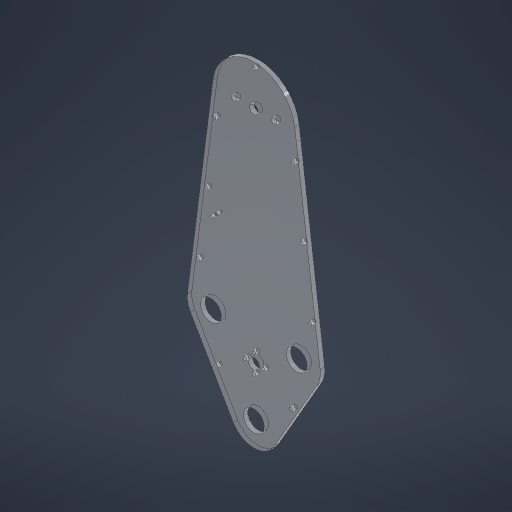
# Autodesk Inventor part: 2ELO
Saved by Autodesk Inventor 2025.2 (Build 292293000, 293)
## iProperties
Created: 2025-05-02
Part Number: 2ELO
Material: Generic
Document SubType Name: Modeling
Designer: Nelson
Density: 1 g/cm^3
Appearance: Polycarbonate - Clear
Author: Nelson
Autodesk Inventor part; units mm, degrees
ref_plane "YZ Plane" through (0, 0, 0) normal (1, 0, 0) x (0, 1, 0)
ref_plane "XZ Plane" through (0, 0, 0) normal (0, 1, 0) x (-1, 0, 0)
ref_plane "XY Plane" through (0, 0, 0) normal (0, 0, 1) x (1, 0, 0)
sketch "Sketch1" plane through (0, 0, 0) normal (0, 0, 1) x (1, 0, 0)
  line L0 (0, 0) -> (0, 200) construction
  arc A0 (37.1934, 204.7857) -> (-37.1934, 204.7857) centre (0, 200) ccw
  line L1 (0, 200) -> (-18.25, 200) construction
  circle A1 centre (-18.25, 200) radius 2.5
  line L2 (0, 200) -> (18.25, 200) construction
  circle A2 centre (18.25, 200) radius 2.5
  circle A3 centre (0, 0) radius 15 construction
  line L3 (37.1934, 204.7857) -> (59.7122, 29.7756)
  line L4 (-37.1934, 204.7857) -> (-59.9286, 28.0941)
  line L5 (48.4528, 117.2807) -> (43.4937, 116.6426) construction
  line L6 (51.1509, 57.1332) -> (35.8365, 176.152) construction
  circle A4 centre (35.8365, 176.152) radius 1.5
  circle A5 centre (51.1509, 57.1332) radius 1.5
  circle A6 centre (43.4937, 116.6426) radius 1.5
  line L7 (0, 237.5) -> (0, 232.5) construction
  circle A7 centre (0, 232.5) radius 1.5
  circle A8 centre (-35.8365, 176.152) radius 1.5
  circle A9 centre (-43.4937, 116.6426) radius 1.5
  circle A10 centre (-51.1509, 57.1332) radius 1.5
  circle A11 centre (0, 200) radius 4
  circle A12 centre (0, 0) radius 45 construction
  circle A13 centre (0, -45) radius 9.5
  circle A14 centre (0, -45) radius 14.5 construction
  circle A15 centre (0, -59.5) radius 2.25 construction
  circle A16 centre (14.5, -45) radius 2.25 construction
  circle A17 centre (0, -30.5) radius 2.25 construction
  circle A18 centre (-14.5, -45) radius 2.25 construction
  circle A19 centre (0, -45) radius 21.5 construction
  circle A20 centre (38.9711, 22.5) radius 21.5 construction
  circle A21 centre (51.5285, 29.75) radius 2.25 construction
  circle A22 centre (46.2211, 9.9426) radius 2.25 construction
  circle A23 centre (31.7211, 35.0574) radius 2.25 construction
  circle A24 centre (26.4138, 15.25) radius 2.25 construction
  circle A25 centre (38.9711, 22.5) radius 9.5
  circle A26 centre (-38.9711, 22.5) radius 21.5 construction
  circle A27 centre (-51.5285, 29.75) radius 2.25 construction
  circle A28 centre (-31.7211, 35.0574) radius 2.25 construction
  circle A29 centre (-46.2211, 9.9426) radius 2.25 construction
  circle A30 centre (-26.4138, 15.25) radius 2.25 construction
  circle A31 centre (-38.9711, 22.5) radius 9.5
  line L8 (-18.6195, -55.75) -> (-57.5907, 11.75)
  line L9 (18.6195, -55.75) -> (57.5907, 11.75)
  line L10 (48.4528, 117.2807) -> (48.4528, 23.0901) construction
  line L11 (59.7122, 29.7756) -> (60.2953, 25.2438)
  line L12 (48.4528, 23.0901) -> (48.4528, -26.9099) construction
  line L13 (48.4528, -26.9099) -> (38.566, -21.2018) construction
  line L14 (38.566, -21.2018) -> (34.2359, -18.7018) construction
  circle A32 centre (34.2359, -18.7018) radius 1.5
  circle A33 centre (-34.2359, -18.7018) radius 1.5
  arc A34 (57.5907, 11.75) -> (60.2953, 25.2438) centre (38.9711, 22.5) ccw
  arc A35 (-60.2953, 25.2438) -> (-57.5907, 11.75) centre (-38.9711, 22.5) ccw
  arc A36 (-18.6195, -55.75) -> (18.6195, -55.75) centre (0, -45) ccw
  line L15 (38.9711, 22.5) -> (53.4711, 22.5) construction
  line L16 (-59.9286, 28.0941) -> (-60.2953, 25.2438)
  circle A37 centre (0, 0) radius 5.1
  line L17 (0, 0) -> (0, -8) construction
  circle A38 centre (0, -8) radius 1.75
  circle A39 centre (8, 0) radius 1.75
  circle A40 centre (0, 8) radius 1.75
  circle A41 centre (-8, 0) radius 1.75
  line L18 (0, 200) -> (0, 135) construction
  line L19 (0, 135) -> (-52.9913, 82.0087) construction
  line L20 (-52.9913, 82.0087) -> (-38.8492, 96.1508) construction
  circle A42 centre (-38.8492, 96.1508) radius 1.1
  line L21 (-38.8492, 96.1508) -> (-33.8994, 101.1006) construction
  circle A43 centre (-33.8994, 101.1006) radius 1.1
  dimension "d84" = 90
  dimension "d86" = 29
  dimension "d58" = 200
  dimension "d59" = 75
  dimension "d60" = 18.25
  dimension "d61" = 5
  dimension "d62" = 30
  dimension "d63" = 5
  dimension "d64" = 120
  dimension "d65" = 3
  dimension "d66" = 3
  dimension "d67" = 3
  dimension "d68" = 5
  dimension "d69" = 3
  dimension "d70" = 8
  dimension "d85" = 19
  dimension "d87" = 4.5
  dimension "d88" = 45
  dimension "d89" = 14.5
  dimension "d90" = 14.5
  dimension "d91" = 360
  dimension "d92" = 43
  dimension "d93" = 360
  dimension "d94" = 94.1906
  dimension "d95" = 50
  dimension "d96" = 5
  dimension "d97" = 3
  dimension "d103" = 10.2
  dimension "d104" = 8
  dimension "d105" = 3.5
  dimension "d108" = 360
  dimension "d110" = 65
  dimension "d111" = 45
  dimension "d112" = 20
  dimension "d113" = 2.2
  dimension "d114" = 7
  dimension "d115" = 2.2
  constraints: 44 end point, 41 centre point, 24 coincident, 15 point on circle, 12 tangent, 7 point on line, 6 symmetric about line, 6 vertical alignment, 4 vertical, 2 concentric, 2 horizontal, 2 horizontal alignment, 2 midpoint, 2 perpendicular, 1 collinear, 1 parallel, 71 other
  measures "d58" distance of L0.start L0.end
  measures "d59" diameter of A0
  measures "d60" distance of L1.start L1.end
  measures "d61" diameter of A1
  measures "d62" diameter of A3
  measures "d63" distance of L5.start L5.end
  measures "d64" distance of L6.start L6.end
  measures "d65" diameter of A4
  measures "d66" diameter of A5
  measures "d67" diameter of A6
  measures "d68" distance of L7.start L7.end
  measures "d69" diameter of A7
  measures "d70" diameter of A11
  measures "d85" diameter of A13
  measures "d87" diameter of A15
  measures "d88" distance of point (0, 0) A13.centre
  measures "d89" distance of A13.centre A15.centre
  measures "d90" distance of A15.centre point (0, -45)
  measures "d92" diameter of A19
  measures "d94" distance of L5.start L10.end
  measures "d95" distance of L10.end L13.start
  measures "d96" distance of L13.end L14.end
  measures "d97" diameter of A32
  measures "d103" diameter of A37
  measures "d104" distance of L17.start L17.end
  measures "d105" diameter of A38
  measures "d110" distance of A11.centre L18.end
  measures "d111" angle of L0 L19
  measures "d112" distance of L19.end L20.end
  measures "d113" diameter of A42
  measures "d114" distance of L21.start L21.end
  measures "d115" diameter of A43
extrude "Extrusion1" add sketch "Sketch1" along normal blind 4
sketch "Sketch2" plane through (0, 0, 4) normal (0, 0, 1) x (1, 0, 0)
  line L0 (0, 0) -> (0, -70) construction
  line L1 (0.05, -69.95) -> (-0.05, -69.95)
  line L2 (-0.05, -69.95) -> (-0.05, -70.05)
  line L3 (-0.05, -70.05) -> (0.05, -70.05)
  line L4 (0.05, -70.05) -> (0.05, -69.95)
  line L5 (0.05, -69.95) -> (-0.05, -70.05) construction
  line L6 (-0.05, -69.95) -> (0.05, -70.05) construction
  dimension "d47" = 70
  dimension "d48" = 0.1
  dimension "d49" = 0.1
  constraints: 14 end point, 2 midpoint, 2 parallel, 1 horizontal, 1 perpendicular, 1 vertical
  measures "d47" distance of L0.start L0.end
  measures "d48" distance of L1.end L2.end
  measures "d49" distance of L1.start L1.end
extrude "Extrusion2" add sketch "Sketch2" along normal blind 0.1
equation "\"d63\" = d101"
equation "\"d65\" = d102"
equation "\"d66\" = d102"
equation "\"d67\" = d102"
equation "\"d68\" = d101"
equation "\"d69\" = d102"
equation "\"d96\" = d101"
equation "\"d97\" = d102"
equation "\"d101\" = 5"
equation "\"d102\" = 3"
body "Solid1"
